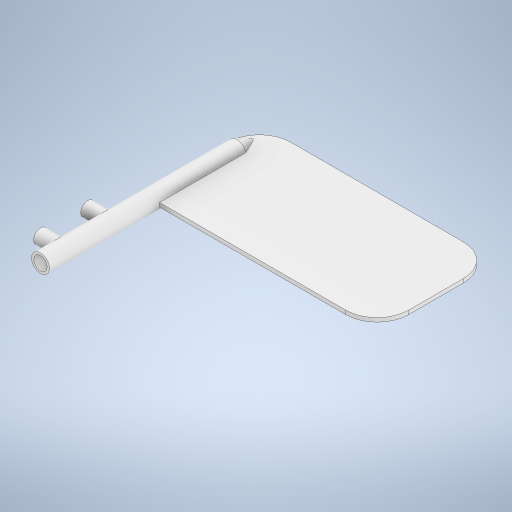
# Autodesk Inventor part: HTW-000692
Saved by Autodesk Inventor 2024.4 (Build 284460000, 460)
## iProperties
Created: 2026-01-12
Part Number: HTW-000692
Material: PVC, hart
Document SubType Name: Modeling
Designer: PC
Density: 1.29 g/cm^3
Appearance: Glatt - Weiß
Description: Ruder
Mass: 311.76 g
Surface Area: 1526.68 cm^2
Volume: 346.785 cm^3
Masse[kg]: 0,312 kg
Author: PC
Autodesk Inventor part; units mm, degrees
ref_plane "YZ Plane" through (0, 0, 0) normal (1, 0, 0) x (0, 1, 0)
ref_plane "XZ Plane" through (0, 0, 0) normal (0, 1, 0) x (-1, 0, 0)
ref_plane "XY Plane" through (0, 0, 0) normal (0, 0, 1) x (1, 0, 0)
sketch "Skizze1" plane through (0, 0, 0) normal (0, 1, 0) x (-1, 0, 0)
  circle A0 centre (0, 0) radius 8.5
  circle A1 centre (0, 0) radius 11.5
  dimension "d0" = 17
  dimension "d1" = 3
  constraints: 2 centre point, 1 coincident
  measures "d0" diameter of A0
  measures "d1" radial gap between concentric circles of A0 A1
extrude "Extrusion1" add sketch "Skizze1" along normal blind 250
sketch "Skizze2" plane through (0, 0, 0) normal (0, 0, 1) x (1, 0, 0)
  line L0 (11.5, 250) -> (-11.5, 250) projected
  line L1 (-11.5, 250) -> (-11.5, 250)
  line L2 (28.5, 290) -> (248.5, 290)
  line L3 (288.5, 250) -> (288.5, 180)
  line L4 (248.5, 140) -> (8.5, 140)
  line L5 (8.5, 250) -> (8.5, 0) projected
  arc A0 (248.5, 140) -> (288.5, 180) centre (248.5, 180) ccw
  arc A1 (288.5, 250) -> (248.5, 290) centre (248.5, 250) ccw
  arc A2 (28.5, 290) -> (-11.5, 250) centre (28.5, 250) ccw
  point P0 (0, 0)
  point P1 (-11.5, 290)
  point P2 (288.5, 290)
  point P3 (288.5, 140)
  dimension "d4" = 40
  dimension "d5" = 300
  dimension "d6" = 150
  dimension "d7" = 40
  constraints: 8 end point, 7 point on line, 6 point on circle, 6 tangent, 3 centre point, 3 perpendicular, 2 equal radius, 1 vertical
  measures "d4" distance of L0.end point (-11.5, 290)
  measures "d5" distance of point (-11.5, 290) point (288.5, 290)
  measures "d6" distance of point (288.5, 290) point (288.5, 140)
  measures "d7" radius of A0
extrude "Extrusion2" add sketch "Skizze2" along normal mid plane 5
sketch "Skizze3" plane through (0, 0, 0) normal (1, 0, 0) x (0, 1, 0)
  line L0 (250, -11.5) -> (250, -2.5) projected
  line L1 (250, -2.5) -> (180, -2.5) projected
  line L2 (250, -2.5) -> (250, -2.5)
  line L3 (250, -2.5) -> (250, -11.5)
  line L4 (-70, 0) -> (420, 0) projected
  line L5 (250, -11.5) -> (270, -2.5)
  line L6 (250, -2.5) -> (290, -2.5) projected
  point P0 (0, 0)
  constraints: 6 end point, 1 horizontal, 1 midpoint, 1 perpendicular
revolve "Umdrehung1" add sketch "Skizze3" angle 360 about axis through (0, -10, 0) along (0, 1, 0)
sketch "Skizze4" plane through (0, 0, 0) normal (1, 0, 0) x (0, 1, 0)
  line L0 (0, 0) -> (30, 0)
  line L1 (30, 0) -> (90, 0)
  circle A0 centre (30, 0) radius 5
  circle A1 centre (90, 0) radius 5
  dimension "d11" = 30
  dimension "d12" = 60
  dimension "d13" = 10
  dimension "d14" = 10
  constraints: 4 end point, 2 centre point, 2 coincident, 1 horizontal, 1 point on line
  measures "d11" distance of L0.start L0.end
  measures "d12" distance of L0.end L1.end
  measures "d13" diameter of A0
  measures "d14" diameter of A1
extrude "Extrusion3" cut sketch "Skizze4" against normal through all
sketch "Skizze5" plane through (0, 0, 0) normal (1, 0, 0) x (0, 1, 0)
  line L0 (0, 0) -> (30, 0)
  circle A0 centre (30, 0) radius 4
  circle A1 centre (30, 0) radius 9
  line L1 (30, 0) -> (90, 0)
  circle A2 centre (90, 0) radius 4
  circle A3 centre (90, 0) radius 9
  dimension "d17" = 30
  dimension "d18" = 8
  dimension "d19" = 5
  dimension "d20" = 60
  dimension "d21" = 8
  dimension "d22" = 5
  constraints: 4 centre point, 4 end point, 2 coincident, 2 horizontal
  measures "d17" distance of L0.start L0.end
  measures "d18" diameter of A0
  measures "d19" radial gap between concentric circles of A0 A1
  measures "d20" distance of L1.start L1.end
  measures "d21" diameter of A2
  measures "d22" radial gap between concentric circles of A2 A3
extrude "Extrusion4" add sketch "Skizze5" against normal blind 30 contours A1 L1 A0 L0 | A3 | L0 A0 L1 A1
sketch "Skizze6" plane through (0, 0, 0) normal (0, -1, 0) x (1, 0, 0)
  circle A0 centre (0, 0) radius 8.5
  dimension "d25" = 17
  constraints: 1 centre point, 1 coincident
  measures "d25" diameter of A0
extrude "Extrusion5" cut sketch "Skizze6" against normal blind 250
thread "Gewinde3" size "M8x1.25" class "6H" standard "ANSI Metric M Profile" length 60
thread "Gewinde4" size "M8x1.25" class "6H" standard "ANSI Metric M Profile" length 60
